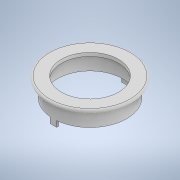
# Autodesk Inventor part: vez-rotate
Saved by Autodesk Inventor 2022 (Build 260153000, 153)
## iProperties
Created: 2022-11-30
Part Number: vez-rotate
Material: Generic
Document SubType Name: Modeling
Designer: matys
Density: 1 g/cm^3
Appearance: Default
Author: matys
Autodesk Inventor part; units mm, degrees
ref_plane "YZ Plane" through (0, 0, 0) normal (1, 0, 0) x (0, 1, 0)
ref_plane "XZ Plane" through (0, 0, 0) normal (0, 1, 0) x (-1, 0, 0)
ref_plane "XY Plane" through (0, 0, 0) normal (0, 0, 1) x (1, 0, 0)
sketch "Sketch1" plane through (0, 0, 0) normal (0, 1, 0) x (-1, 0, 0)
  circle A0 centre (0, 0) radius 28
  line L0 (28, 0) -> (31.5, 0)
  circle A1 centre (0, 0) radius 31.5
  circle A2 centre (0, 0) radius 31.5
  circle A3 centre (0, 0) radius 31.5
  dimension "d0" = 56
  dimension "d1" = 3.5
  constraints: 4 coincident, 4 horizontal alignment, 2 end point, 1 horizontal, 8 other
  measures "d1" distance of L0.start L0.end
extrude "Extrusion1" add sketch "Sketch1" along normal blind 13.25
sketch "Sketch2" plane through (0, 13.25, 0) normal (0, 1, 0) x (1, 0, 0)
  circle A0 centre (0, 0) radius 28 projected
  line L0 (0, -28) -> (0, -24.5)
  line L1 (0, -24.5) -> (0, -31.5)
  circle A1 centre (0, 0) radius 31.5 projected
  line L2 (0, -31.5) -> (0, -36)
  circle A2 centre (0, 0) radius 24.5
  circle A3 centre (0, 0) radius 36
  dimension "d4" = 3.5
  dimension "d5" = 4.5
  constraints: 6 end point, 4 vertical alignment, 2 coincident, 2 point on line, 1 vertical, 6 other
  measures "d4" distance of L0.start L0.end
  measures "d5" distance of L1.end L2.end
extrude "Extrusion2" add sketch "Sketch2" along normal blind 3 contours A0 | A1 | A3
sketch "Sketch3" plane through (0, 0, 0) normal (0, -1, 0) x (1, 0, 0)
  circle A0 centre (0, 0) radius 31.5 projected
  line L0 (0.0291, 31.5) -> (0.0291, -31.5)
  line L1 (2.8791, 31.3681) -> (2.8791, -35.492)
  line L2 (-2.8209, 31.3734) -> (-2.8209, -35.492)
  circle A1 centre (0, 0) radius 31.5
  circle A2 centre (0, 0) radius 30
  point P0 (2.8791, 29.8615)
  point P1 (2.8791, 31.3681)
  point P2 (-2.8209, 31.3734)
  point P3 (-2.8209, 29.8671)
  point P4 (2.8791, -29.8615)
  point P5 (-2.8209, -29.8671)
  point P6 (-2.8209, -31.3734)
  point P7 (2.8791, -31.3681)
  dimension "d8" = 2.85
  dimension "d9" = 2.85
  constraints: 6 end point, 4 point on circle, 2 centre point, 2 coincident, 2 parallel, 1 concentric, 1 vertical
  measures "d8" distance between parallel lines of L0 L1
  measures "d9" distance between parallel lines of L0 L2
extrude "Extrusion3" add sketch "Sketch3" along normal blind 5 contours L1 A2 L0 A0 | A0 L0 A2 L1 | L0 A2 L2 A0 | A0 L2 A2 L0
fillet "Fillet1" radius 1.5 2 edges at (-36, 13.25, 0) (-36, 16.25, 0)
body "Solid1"
